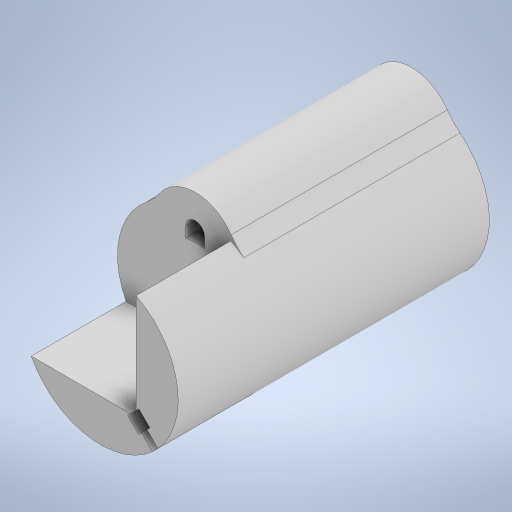
# Autodesk Inventor part: LandingFoot1
Saved by Autodesk Inventor 2023 (Build 270158000, 158)
## iProperties
Created: 2023-01-25
Part Number: LandingFoot1
Material: Generic
Document SubType Name: Modeling
Designer: chase
Density: 1 g/cm^3
Appearance: Default
Author: chase
Autodesk Inventor part; units mm, degrees
ref_plane "YZ Plane" through (0, 0, 0) normal (1, 0, 0) x (0, 1, 0)
ref_plane "XZ Plane" through (0, 0, 0) normal (0, 1, 0) x (-1, 0, 0)
ref_plane "XY Plane" through (0, 0, 0) normal (0, 0, 1) x (1, 0, 0)
sketch "Sketch1" plane through (0, 0, 0) normal (0, 0, 1) x (1, 0, 0)
  circle A0 centre (0, 0) radius 12.5
  dimension "d0" = 25
  constraints: 1 centre point
  measures "d0" diameter of A0
extrude "Extrusion1" add sketch "Sketch1" against normal blind 50
sketch "Sketch2" plane through (0, 0, 0) normal (0, 0, 1) x (1, 0, 0)
  circle A0 centre (0, 0) radius 12.5 projected
  line L0 (0, 12.5) -> (0, 0) construction
  line L1 (0, 0) -> (8.8388, -8.8388) construction
  line L2 (4.4194, -2.6517) -> (9.7227, -7.955)
  line L3 (9.7227, -7.955) -> (7.955, -9.7227)
  line L4 (7.955, -9.7227) -> (2.6517, -4.4194)
  line L5 (4.4194, -2.6517) -> (2.6517, -4.4194)
  line L6 (9.7227, -7.955) -> (7.955, -9.7227)
  line L7 (7.955, -6.1872) -> (6.1872, -7.955)
  line L8 (6.1872, -4.4194) -> (4.4194, -6.1872)
  line L9 (5.374, -4.5255) -> (4.5255, -5.374)
  line L10 (4.4194, -2.6517) -> (2.6517, -4.4194)
  line L11 (5.2679, -4.6315) -> (3.8537, -3.2173)
  line L12 (4.9497, -4.9497) -> (3.5355, -3.5355)
  line L13 (4.6315, -5.2679) -> (3.2173, -3.8537)
  line L14 (9.2631, -8.4146) -> (7.4953, -6.6468)
  line L15 (5.7276, -4.879) -> (5.374, -4.5255)
  line L16 (8.4146, -9.2631) -> (6.6468, -7.4953)
  line L17 (4.879, -5.7276) -> (4.5255, -5.374)
  line L18 (4.879, -5.7276) -> (-11.1106, -5.7276)
  line L19 (5.7276, -4.879) -> (5.7276, 11.1106)
  point P0 (5.7276, -3.9598)
  point P1 (3.9598, -5.7276)
  dimension "d12" = 135
  dimension "d14" = 7.5
  dimension "d16" = 7.5
  dimension "d18" = 2.5
  dimension "d19" = 2.5
  dimension "d20" = 0.5
  dimension "d25" = 0.45
  dimension "d26" = 0.45
  dimension "d27" = 1.2
  constraints: 40 end point, 6 parallel, 6 point on line, 4 point on circle, 2 perpendicular, 1 collinear, 1 horizontal, 1 tangent, 1 vertical
  measures "d12" angle of L1 L0
  measures "d14" distance of L2.start L2.end
  measures "d16" distance of L3.end L4.end
  measures "d18" distance between parallel lines of L3 L7
  measures "d19" distance between parallel lines of L7 L8
  measures "d20" distance between parallel lines of L8 L9
  measures "d25" distance between parallel lines of L11 L12
  measures "d26" distance between parallel lines of L12 L13
  measures "d27" distance between parallel lines of L16 L14
extrude "Extrusion2" cut sketch "Sketch2" against normal blind 15.24 contours L19 L2 L5 L4 L18 A0 | L19 L15 L9 L11 L5 L2 | L14 L3 A0 | A0 L16 L7 L14 | L7 L4 L8 L2 | L4 L5 L13 L9 L17 L18 | L8 L17 L9 L15 | L3 L16 A0 | L11 L9 L12 L5 | L5 L12 L9 L13
sketch "Sketch3" plane through (0, 0, -50) normal (0, 0, -1) x (-1, 0, 0)
  circle A0 centre (0, 0) radius 8.075
  circle A1 centre (0, 9.575) radius 1.5
  line L0 (-1.5, 9.575) -> (-1.5, 7.9345)
  line L1 (1.5, 9.575) -> (1.5, 7.9345)
  dimension "d30" = 16.15
  dimension "d33" = 3
  constraints: 4 end point, 4 point on circle, 2 centre point, 1 coincident, 1 parallel, 1 tangent, 1 vertical
  measures "d30" diameter of A0
  measures "d33" diameter of A1
extrude "Extrusion3" cut sketch "Sketch3" against normal blind 25.4 contours A0
extrude "Extrusion4" cut sketch "Sketch3" against normal through all contours A0 A1 L1 | L0 A1 A0 | A1
sketch "Sketch4" plane through (0, 0, -50) normal (0, 0, -1) x (-1, 0, 0)
  arc A0 (6.4283, 10.7204) -> (-6.4283, 10.7204) centre (0, 8.075) ccw
  arc A1 (1.5, 7.9345) -> (-1.5, 7.9345) centre (0, 0) ccw projected
  circle A2 centre (0, 0) radius 12.5 projected
  point P0 (0, 8.075)
  dimension "d37" = 12.8567
  dimension "d38" = 6.4283
  constraints: 6 point on circle, 1 centre point
  measures "d37" distance of A0.start A0.end
  measures "d38" horizontal distance of A0.start point (0, 8.075)
extrude "Extrusion5" add sketch "Sketch4" against normal up to surface (34.76 mm away) contours A2 A0
fillet "Fillet1" radius 10 2 edges at (-6.4283, 10.7204, -32.62) (6.4283, 10.7204, -32.62)
equation "\"d38\" = 0.5 * d37"
body "Solid1"
